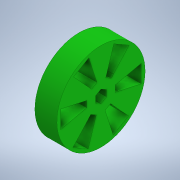
# Autodesk Inventor part: part_4 in. Compliance Wheel
Saved by Autodesk Inventor 2021.1 (Build 251245000, 245)
## iProperties
Created: 2020-01-14
Part Number: part_4 in. Compliance Wheel
Material: ABS Plastic
Document SubType Name: Modeling
Designer: woodn
Density: 1.06 g/cm^3
Appearance: Dark Green
Author: woodn
Autodesk Inventor part; units mm, degrees
ref_plane "YZ Plane" through (0, 0, 0) normal (1, 0, 0) x (0, 1, 0)
ref_plane "XZ Plane" through (0, 0, 0) normal (0, 1, 0) x (-1, 0, 0)
ref_plane "XY Plane" through (0, 0, 0) normal (0, 0, 1) x (1, 0, 0)
sketch "Sketch1" plane through (0, 0, 0) normal (1, 0, 0) x (0, 1, 0)
  circle A0 centre (0, 0) radius 50.8
  dimension "d16" = 101.6
  constraints: 1 centre point, 1 coincident
  measures "d16" diameter of A0
extrude "Extrusion1" add sketch "Sketch1" along normal blind 25.4
sketch "Sketch2" plane through (25.4, 0, 0) normal (1, 0, 0) x (0, 0, -1)
  circle A0 centre (0, 0) radius 50.8
  circle A1 centre (0, 0) radius 25.4
  line L0 (6.35, 3.6662) -> (6.35, -3.6662)
  line L1 (6.35, -3.6662) -> (0, -7.3323)
  line L2 (0, -7.3323) -> (-6.35, -3.6662)
  line L3 (-6.35, -3.6662) -> (-6.35, 3.6662)
  line L4 (-6.35, 3.6662) -> (0, 7.3323)
  line L5 (0, 7.3323) -> (6.35, 3.6662)
  circle A2 centre (0, 0) radius 44.45
  line L6 (0, 0) -> (-11.3174, 49.5233)
  circle A3 centre (0, 0) radius 50.8 projected
  line L7 (0, 0) -> (10.4532, 49.7129)
  arc A4 (9.1466, 43.4988) -> (-9.9027, 43.3329) centre (0, 0) ccw
  point P0 (5.2266, 24.8564)
  point P1 (-5.6587, 24.7616)
  dimension "d3" = 25.4
  dimension "d4" = 6.35
  dimension "d5" = 0
  dimension "d8" = 6.35
  dimension "d9" = 19.05
  dimension "d10" = 0
  constraints: 16 end point, 6 point on circle, 4 centre point, 2 coincident, 2 point on line, 14 other
  measures "d3" radial gap between concentric circles of A0 A1
  measures "d4" distance from line of point (0, 0) L5
  measures "d5" horizontal distance of point (0, 0) L4.end
  measures "d8" radial gap between concentric circles of A0 A2
  measures "d9" distance of A2.start A2.end
  measures "d10" distance of point (0, 0) A4.centre
extrude "Extrusion4" cut sketch "Sketch2" against normal through all contours L7 L6 L4 L5 | L5 L0 L1 L2 L3 L4 L6 L7
sketch "Sketch3" plane through (25.4, 0, 0) normal (1, 0, 0) x (0, 0, -1)
  circle A0 centre (0, 0) radius 50.8 projected
  line L0 (-46.4628, -9.6079) -> (-46.4628, 9.6097)
  line L1 (-16.4289, -3.168) -> (-41.9244, -8.8202)
  line L2 (-42.0194, 9.6834) -> (-20.1547, 4.9235)
  line L3 (-16.4289, 4.1621) -> (-16.4289, -3.168)
  line L4 (-16.4289, 4.1621) -> (-20.1547, 4.9235)
  line L5 (-42.0194, 9.6834) -> (-46.4628, 10.6507)
  line L6 (-46.4628, 10.6507) -> (-46.4628, 9.6097)
  line L7 (-41.9244, -8.8202) -> (-46.4628, -9.8264)
  line L8 (-46.4628, -9.8264) -> (-46.4628, -9.6079)
  constraints: 18 end point, 4 vertical
extrude "Extrusion5" cut sketch "Sketch3" against normal through all contours L0 L6 L5 L2 L4 L3 L1 L7 L8
pattern_circular "Circular Pattern2" count 6 over 360 about axis through (0, 0, 0) along (1, 0, 0) of "Extrusion5"
body "Solid1"
